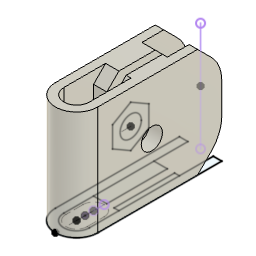
Blackhawk Holster Belt Spacer v6 (Autodesk Fusion 360 design; units mm, degrees)
Autodesk Fusion 360 part; units mm, degrees
sketch "Sketch1" plane through (0, 0, 0) normal (0, 0, 1) x (1, 0, 0)
  line L0 (1.75, -1.4) -> (1.75, 1.4) construction
  arc A0 (1.75, 1.4) -> (-1.75, 1.4) centre (0, 1.4) ccw construction
  line L1 (-1.75, 1.4) -> (-1.75, -1.4) construction
  arc A1 (-1.75, -1.4) -> (1.75, -1.4) centre (0, -1.4) ccw construction
  line L2 (0, -1.4) -> (0, 1.4) construction
  line L3 (0, 3.15) -> (0, -3.15) construction
  line L4 (-2.1, 19.1) -> (-2.1, -1.4)
  arc A2 (-2.1, -1.4) -> (2.1, -1.4) centre (0, -1.4) ccw
  line L5 (2.1, -1.4) -> (2.1, 19.1)
  line L6 (-2.1, 19.1) -> (-3.5, 19.1)
  line L7 (-3.5, 19.1) -> (-3.5, -1.4)
  line L8 (2.1, 19.1) -> (3.5, 19.1)
  line L9 (3.5, 19.1) -> (3.5, -1.4)
  arc A3 (-3.5, -1.4) -> (3.5, -1.4) centre (0, -1.4) ccw
  line L10 (2.1, 13.5) -> (1.3, 13.5)
  line L11 (1.3, 13.5) -> (1.3, 3.5)
  line L12 (1.3, 3.5) -> (2.1, 3.5)
  line L13 (-2.1, 13.5) -> (0.1, 13.5)
  line L14 (0.1, 13.5) -> (0.1, 3.5)
  line L15 (0.1, 3.5) -> (-2.1, 3.5)
  point P0 (0, -4.9)
  dimension "d1" = 3.5
  dimension "d2" = 6.3
  dimension "d12" = 24
  dimension "d14" = 2.1
  dimension "d15" = 1.4
  dimension "d16" = 10
  dimension "d17" = 3.5
  dimension "d25" = 2.2
  dimension "d26" = 0.8
  constraint tangent L0 A0
  constraint tangent A0 L1
  constraint parallel L0 L1
  constraint tangent L1 A1
  constraint tangent L0 A1
  constraint vertical L2
  constraint midpoint A0 L3.start
  constraint midpoint A1 L3.end
  constraint parallel L1 L3
  constraint midpoint L2 origin
  constraint vertical L4
  constraint tangent L4 A2
  constraint vertical L5
  constraint tangent A2 L5
  constraint coincident A1.centre L2.start
  constraint perpendicular L4 L6
  constraint perpendicular L5 L8
  constraint coincident L9.end A3.end
  constraint tangent L7 A3
  constraint vertical L9
  constraint vertical L7
  constraint tangent L9 A3
  constraint collinear L6 L8
  constraint midpoint A3 P0
  constraint coincident L5 L10.start
  constraint perpendicular L5 L10
  constraint perpendicular L10 L11
  constraint coincident L5 L12.end
  constraint perpendicular L5 L12
  constraint coincident L4 L13.start
  constraint perpendicular L4 L13
  constraint perpendicular L12 L14
  constraint coincident L4 L15.end
  constraint perpendicular L4 L15
  constraint collinear L10 L13
  constraint collinear L12 L15
  measures "d1" distance of L0 L1
  measures "d2" distance of L3.start L3.end
  measures "d12" distance of L8 P0
  measures "d14" radius of A2
  measures "d15" distance of A2 A3
  measures "d16" distance of L13.end L14.end
  measures "d17" distance of origin L12
  measures "d25" distance of L13.start L13.end
  measures "d26" distance of L10.start L10.end
extrude "Extrude1" add sketch "Sketch1" along normal blind 18
sketch "Sketch2" plane through (0, 0, 0) normal (1, 0, 0) x (0, 1, 0)
  line L0 (19.1, 0) -> (19.1, 18)
  circle A0 centre (7.55, 9) radius 1.75
  line L1 (3.15, 0) -> (1.4, 0)
  line L2 (7.55, 9) -> (5.8, 9) construction
  line L3 (10.55, 10.7321) -> (7.55, 12.4641)
  line L4 (7.55, 12.4641) -> (4.55, 10.7321)
  line L5 (4.55, 10.7321) -> (4.55, 7.2679)
  line L6 (4.55, 7.2679) -> (7.55, 5.5359)
  line L7 (7.55, 5.5359) -> (10.55, 7.2679)
  line L8 (10.55, 7.2679) -> (10.55, 10.7321)
  point P0 (19.1, 9)
  point P1 (3.15, 0)
  point P2 (7.55, 9)
  dimension "d7" = 3.5
  dimension "d20" = 6
  dimension "d24" = 1.4
  constraint midpoint L0 P0
  constraint horizontal P2 P0
  constraint coincident P2 A0.centre
  constraint coincident A0 L2.end
  constraint horizontal L2
  constraint vertical L8
  measures "d7" diameter of A0
  measures "d20" distance of L5 L8
  measures "d24" distance of P1 L5
extrude "Extrude2" cut sketch "Sketch2" along normal mid plane 14 contours A0
chamfer "Chamfer1" distance 4 angle 45 4 edges at (2.8, 19.1, 0) (-2.8, 19.1, 0) (2.8, 19.1, 18) (-2.8, 19.1, 18)
fillet "Fillet1" radius 6 4 edges at (2.8, 19.1, 4) (2.8, 19.1, 14) (-2.8, 19.1, 4) (-2.8, 19.1, 14)
extrude "Extrude3" cut sketch "Sketch2" along normal blind 2 from surface at -3.5
chamfer "Chamfer2" distance 2 angle 45 8 edges at (-1, 13.5, 18) (-1, 3.5, 18) (1.7, 13.5, 18) (1.7, 3.5, 18) (1.7, 13.5, 0) (-1, 13.5, 0) (1.7, 3.5, 0) (-1, 3.5, 0)
named bodies: "Belt Spacer"
